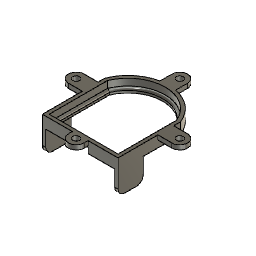
AMT103_MountingFrame v2 (Autodesk Fusion 360 design; units mm, degrees)
Autodesk Fusion 360 part; units mm, degrees
sketch "Sensor_AMT103" plane through (0, 0, 0) normal (0, 0, 1) x (1, 0, 0) in component "SensorMount"
  line L0 (-14.3, -18.71) -> (14.3, -18.71)
  arc A0 (14.3, 5.98) -> (-14.3, 5.98) centre (0, 0) ccw
  line L1 (14.3, 5.98) -> (14.3, -18.71)
  line L2 (-14.3, 5.98) -> (-14.3, -18.71)
  line L3 (0, 0) -> (26.3569, 0) construction
  line L4 (0, 0) -> (0, 31) construction
  circle A1 centre (0, 0) radius 23 construction
  circle A2 centre (23, 0) radius 1.5
  circle A3 centre (0, 23) radius 1.5
  circle A4 centre (-23, 0) radius 1.5
  circle A5 centre (0, -23) radius 1.5
  line L5 (23, -3.5) -> (16.8, -3.5)
  line L6 (-23, -3.5) -> (-16.8, -3.5)
  line L7 (-23, 3.5) -> (-16.8, 3.5)
  line L8 (3.5, -23) -> (3.5, -21.21)
  line L9 (-3.5, -23) -> (-3.5, -21.21)
  line L10 (-3.5, 23) -> (-3.5, 17.6564)
  line L11 (3.5, 23) -> (3.5, 17.6564)
  arc A6 (-3.4899, -22.7337) -> (3.4899, -22.7337) centre (0, -23) ccw
  arc A7 (-22.7337, 3.4899) -> (-22.7337, -3.4899) centre (-23, 0) ccw
  arc A8 (22.7337, -3.4899) -> (22.7337, 3.4899) centre (23, 0) ccw
  line L12 (23, 3.5) -> (16.8, 3.5)
  arc A9 (3.4899, 22.7337) -> (-3.4899, 22.7337) centre (0, 23) ccw
  line L13 (15.3, 6.1774) -> (15.3, -19.71)
  line L14 (-15.3, -19.71) -> (15.3, -19.71)
  line L15 (-15.3, 6.1774) -> (-15.3, -19.71)
  arc A10 (15.3, 6.1774) -> (-15.3, 6.1774) centre (0, 0) ccw
  line L16 (16.8, 6.4622) -> (16.8, -21.21)
  line L17 (-16.8, -21.21) -> (16.8, -21.21)
  line L18 (-16.8, 6.4622) -> (-16.8, -21.21)
  arc A11 (16.8, 6.4622) -> (-16.8, 6.4622) centre (0, 0) ccw
  line L19 (30, -10) -> (-28.5666, -10) construction
  line L20 (16.8, -10) -> (15.3, -10)
  line L21 (-15.3, -10) -> (-16.8, -10)
  line L22 (-15.3, -19.71) -> (-15.3, -21.21)
  line L23 (15.3, -19.71) -> (15.3, -21.21)
  line L24 (3.5, -21.21) -> (3.5, -18.71)
  line L25 (-3.5, -21.21) -> (-3.5, -18.71)
  point P0 (33, 0)
  point P1 (0, 15.5)
  dimension "d539" = 15.5
  dimension "d540" = 14.3
  dimension "d541" = 14.3
  dimension "d544" = 34.21
  dimension "d545" = 46
  dimension "d546" = 3
  dimension "d548" = 360
  dimension "d549" = 1
  dimension "d550" = 2.5
  dimension "d551" = 7
  constraint vertical L1
  constraint vertical L2
  constraint horizontal L0
  constraint coincident A0.centre L3.start
  constraint horizontal L3
  constraint coincident A0.centre L3
  constraint coincident P1 A0
  constraint perpendicular L3 L4
  constraint coincident P1 L4
  constraint coincident A1 A2.centre
  constraint coincident L3 A2.centre
  constraint concentric A2 A8
  constraint perpendicular L1 L12
  constraint perpendicular L1 L5
  constraint tangent A8 L12
  constraint tangent L5 A8
  constraint coincident L12.start A8
  constraint coincident L5.start A8
  constraint coincident L10.end A11
  constraint coincident L11.end A11
  constraint coincident L7.end L18
  constraint coincident L6.end L18
  constraint coincident L8.end L17
  constraint coincident L9.end L17
  constraint coincident A1 A6.end
  constraint coincident A1 A6.start
  constraint coincident A1 A7.end
  constraint coincident A1 A7.start
  constraint coincident A1 A8.end
  constraint coincident A1 A8.start
  constraint coincident L5.end L16
  constraint coincident L12.end L16
  constraint coincident A1 A9.start
  constraint coincident A1 A9.end
  constraint perpendicular L18 L19
  constraint coincident L19 L20.start
  constraint coincident L16 L20.start
  constraint coincident L19 L20.end
  constraint coincident L13 L20.end
  constraint coincident L19 L21.start
  constraint coincident L15 L21.start
  constraint coincident L19 L21.end
  constraint coincident L18 L21.end
  constraint coincident L17 L22.end
  constraint perpendicular L17 L22
  constraint coincident L17 L23.end
  constraint perpendicular L17 L23
  constraint coincident L0 L24.end
  constraint perpendicular L0 L24
  constraint coincident L0 L25.end
  constraint perpendicular L0 L25
  measures "d539" radius of A0
  measures "d540" distance of A0.centre L1
  measures "d541" distance of A0.centre L2
  measures "d544" distance of P1 L0
  measures "d545" diameter of A1
  measures "d546" diameter of A2
  measures "d551" diameter of A8
extrude "Extrude6" add sketch "Sensor_AMT103" against normal blind 2 contours L14 L17 L22 L25 | L14 L17 L24 L25 | L14 L17 L23 L24 | L15 L17 L18 L21 L22 | L8 L9 A6 L17 | L13 L16 L17 L20 L23 | L13 L15 A10 L16 L18 A11 L20 L21 | L6 L7 A7 L18 | L5 A8 L12 L16 | L10 L11 A9 A11 in component "SensorMount"
extrude "Extrude7" add sketch "Sensor_AMT103" against normal blind 5 contours L14 L17 L22 L25 | L14 L17 L23 L24 | L15 L17 L18 L21 L22 | L13 L16 L17 L20 L23 | L13 L15 A10 L16 L18 A11 L20 L21 in component "SensorMount"
extrude "Extrude8" add sketch "Sensor_AMT103" along normal blind -5 and the other way blind 3 contours L0 A0 L1 L2 L13 L14 L15 A10 L24 L25 in component "SensorMount"
extrude "Extrude10" add sketch "Sensor_AMT103" against normal blind 15 contours L15 L17 L18 L21 L22 | L13 L16 L17 L20 L23 in component "SensorMount"
fillet "Fillet1" radius 3 4 edges at (16.05, -10, -15) (-16.05, -10, -15) (-16.05, -21.21, -15) (16.05, -21.21, -15) in component "SensorMount"
fillet "Fillet4" radius 1 5 edges at (0, 15.5, -3) (-14.3, -6.365, -3) (14.3, -6.365, -3) (-8.9, -18.71, -3) (8.9, -18.71, -3) in component "SensorMount"
fillet "Fillet5" radius 1 2 edges at (-3.5, -20.46, -2) (3.5, -20.46, -2) in component "SensorMount"
component "Sensor" placed x (1, 0, 0) y (0, 1, 0) z (0, 0, 1) at (0, 0, 0)
component "SensorMount" placed x (1, 0, 0) y (0, 1, 0) z (0, 0, 1) at (0, 0, 0) in component "Sensor"
equation "d64_1 = ( 15.5 * 2 ) * 1 mm"
equation "d65_1 = ( 28.77 / 2 ) * 1 mm"
equation "MotorHeight = 42 mm"
equation "d540 = ( 28.6 / 2 ) * 1 mm"
equation "d541 = ( 28.6 / 2 ) * 1 mm"
equation "Bottom = MotorHeight + FrontMotorDepth + 5 mm"
equation "FrontMotorDepth = 8 mm"
named bodies: "AMT103_MountingFrame"
